Autodesk Fusion 360 part; units mm, degrees
(part 4 of 4)
  line L740 (15.875, 67.5068) -> (19.375, 69.5275)
  line L741 (28.375, 73.569) -> (24.875, 75.5897)
  line L742 (12.375, 69.5275) -> (15.875, 67.5068)
  line L743 (20.375, 59.7125) -> (23.875, 61.7333)
  line L744 (29.375, 67.7955) -> (25.875, 65.7747)
  line L745 (21.375, 73.569) -> (21.375, 69.5275)
  line L746 (16.875, 61.7333) -> (20.375, 59.7125)
  line L747 (25.875, 61.7333) -> (29.375, 59.7125)
  line L748 (25.875, 65.7747) -> (25.875, 61.7333)
  line L749 (23.875, 61.7333) -> (23.875, 65.7747)
  line L750 (16.875, 65.7747) -> (16.875, 61.7333)
  line L751 (32.875, 61.7333) -> (32.875, 65.7747)
  line L752 (15.875, 75.5897) -> (12.375, 73.569)
  line L753 (32.875, 65.7747) -> (29.375, 67.7955)
  line L754 (37.375, 73.569) -> (33.875, 75.5897)
  line L755 (46.375, 69.5275) -> (46.375, 73.569)
  line L756 (42.875, 75.5897) -> (39.375, 73.569)
  line L757 (39.375, 69.5275) -> (42.875, 67.5068)
  line L758 (41.875, 65.7747) -> (38.375, 67.7955)
  line L759 (37.375, 69.5275) -> (37.375, 73.569)
  line L760 (47.375, 59.7125) -> (50.875, 61.7333)
  line L761 (30.375, 73.569) -> (30.375, 69.5275)
  line L762 (42.875, 67.5068) -> (46.375, 69.5275)
  line L763 (38.375, 67.7955) -> (34.875, 65.7747)
  line L764 (33.875, 67.5068) -> (37.375, 69.5275)
  line L765 (46.375, 73.569) -> (42.875, 75.5897)
  line L766 (30.375, 69.5275) -> (33.875, 67.5068)
  line L767 (38.375, 59.7125) -> (41.875, 61.7333)
  line L768 (47.375, 67.7955) -> (43.875, 65.7747)
  line L769 (39.375, 73.569) -> (39.375, 69.5275)
  line L770 (34.875, 61.7333) -> (38.375, 59.7125)
  line L771 (43.875, 61.7333) -> (47.375, 59.7125)
  line L772 (43.875, 65.7747) -> (43.875, 61.7333)
  line L773 (41.875, 61.7333) -> (41.875, 65.7747)
  line L774 (34.875, 65.7747) -> (34.875, 61.7333)
  line L775 (50.875, 61.7333) -> (50.875, 65.7747)
  line L776 (33.875, 75.5897) -> (30.375, 73.569)
  line L777 (50.875, 65.7747) -> (47.375, 67.7955)
  line L778 (55.375, 73.569) -> (51.875, 75.5897)
  line L779 (64.375, 69.5275) -> (64.375, 73.569)
  line L780 (60.875, 75.5897) -> (57.375, 73.569)
  line L781 (57.375, 69.5275) -> (60.875, 67.5068)
  line L782 (59.875, 65.7747) -> (56.375, 67.7955)
  line L783 (55.375, 69.5275) -> (55.375, 73.569)
  line L784 (65.375, 59.7125) -> (68.875, 61.7333)
  line L785 (48.375, 73.569) -> (48.375, 69.5275)
  line L786 (60.875, 67.5068) -> (64.375, 69.5275)
  line L787 (56.375, 67.7955) -> (52.875, 65.7747)
  line L788 (51.875, 67.5068) -> (55.375, 69.5275)
  line L789 (64.375, 73.569) -> (60.875, 75.5897)
  line L790 (48.375, 69.5275) -> (51.875, 67.5068)
  line L791 (56.375, 59.7125) -> (59.875, 61.7333)
  line L792 (65.375, 67.7955) -> (61.875, 65.7747)
  line L793 (57.375, 73.569) -> (57.375, 69.5275)
  line L794 (52.875, 61.7333) -> (56.375, 59.7125)
  line L795 (61.875, 61.7333) -> (65.375, 59.7125)
  line L796 (61.875, 65.7747) -> (61.875, 61.7333)
  line L797 (59.875, 61.7333) -> (59.875, 65.7747)
  line L798 (52.875, 65.7747) -> (52.875, 61.7333)
  line L799 (68.875, 61.7333) -> (68.875, 65.7747)
  line L800 (51.875, 75.5897) -> (48.375, 73.569)
  line L801 (68.875, 65.7747) -> (65.375, 67.7955)
  line L802 (73.375, 73.569) -> (69.875, 75.5897)
  line L803 (82.375, 69.5275) -> (82.375, 73.569)
  line L804 (78.875, 75.5897) -> (75.375, 73.569)
  line L805 (75.375, 69.5275) -> (78.875, 67.5068)
  line L806 (77.875, 65.7747) -> (74.375, 67.7955)
  line L807 (73.375, 69.5275) -> (73.375, 73.569)
  line L808 (83.375, 59.7125) -> (86.875, 61.7333)
  line L809 (66.375, 73.569) -> (66.375, 69.5275)
  line L810 (78.875, 67.5068) -> (82.375, 69.5275)
  line L811 (74.375, 67.7955) -> (70.875, 65.7747)
  line L812 (69.875, 67.5068) -> (73.375, 69.5275)
  line L813 (82.375, 73.569) -> (78.875, 75.5897)
  line L814 (66.375, 69.5275) -> (69.875, 67.5068)
  line L815 (74.375, 59.7125) -> (77.875, 61.7333)
  line L816 (83.375, 67.7955) -> (79.875, 65.7747)
  line L817 (75.375, 73.569) -> (75.375, 69.5275)
  line L818 (70.875, 61.7333) -> (74.375, 59.7125)
  line L819 (79.875, 61.7333) -> (83.375, 59.7125)
  line L820 (79.875, 65.7747) -> (79.875, 61.7333)
  line L821 (77.875, 61.7333) -> (77.875, 65.7747)
  line L822 (70.875, 65.7747) -> (70.875, 61.7333)
  line L823 (86.875, 61.7333) -> (86.875, 65.7747)
  line L824 (69.875, 75.5897) -> (66.375, 73.569)
  line L825 (86.875, 65.7747) -> (83.375, 67.7955)
  line L826 (91.375, 73.569) -> (87.875, 75.5897)
  line L827 (100.375, 69.5275) -> (100.375, 73.569)
  line L828 (96.875, 75.5897) -> (93.375, 73.569)
  line L829 (93.375, 69.5275) -> (96.875, 67.5068)
  line L830 (95.875, 65.7747) -> (92.375, 67.7955)
  line L831 (91.375, 69.5275) -> (91.375, 73.569)
  line L832 (101.375, 59.7125) -> (104.875, 61.7333)
  line L833 (84.375, 73.569) -> (84.375, 69.5275)
  line L834 (96.875, 67.5068) -> (100.375, 69.5275)
  line L835 (92.375, 67.7955) -> (88.875, 65.7747)
  line L836 (87.875, 67.5068) -> (91.375, 69.5275)
  line L837 (100.375, 73.569) -> (96.875, 75.5897)
  line L838 (84.375, 69.5275) -> (87.875, 67.5068)
  line L839 (92.375, 59.7125) -> (95.875, 61.7333)
  line L840 (101.375, 67.7955) -> (97.875, 65.7747)
  line L841 (93.375, 73.569) -> (93.375, 69.5275)
  line L842 (88.875, 61.7333) -> (92.375, 59.7125)
  line L843 (97.875, 61.7333) -> (101.375, 59.7125)
  line L844 (97.875, 65.7747) -> (97.875, 61.7333)
  line L845 (95.875, 61.7333) -> (95.875, 65.7747)
  line L846 (88.875, 65.7747) -> (88.875, 61.7333)
  line L847 (104.875, 61.7333) -> (104.875, 65.7747)
  line L848 (87.875, 75.5897) -> (84.375, 73.569)
  line L849 (104.875, 65.7747) -> (101.375, 67.7955)
  line L850 (109.375, 73.569) -> (105.875, 75.5897)
  line L851 (118.375, 69.5275) -> (118.375, 73.569)
  line L852 (114.875, 75.5897) -> (111.375, 73.569)
  line L853 (111.375, 69.5275) -> (114.875, 67.5068)
  line L854 (113.875, 65.7747) -> (110.375, 67.7955)
  line L855 (109.375, 69.5275) -> (109.375, 73.569)
  line L856 (119.375, 59.7125) -> (122.875, 61.7333)
  line L857 (102.375, 73.569) -> (102.375, 69.5275)
  line L858 (114.875, 67.5068) -> (118.375, 69.5275)
  line L859 (110.375, 67.7955) -> (106.875, 65.7747)
  line L860 (105.875, 67.5068) -> (109.375, 69.5275)
  line L861 (118.375, 73.569) -> (114.875, 75.5897)
  line L862 (102.375, 69.5275) -> (105.875, 67.5068)
  line L863 (110.375, 59.7125) -> (113.875, 61.7333)
  line L864 (119.375, 67.7955) -> (115.875, 65.7747)
  line L865 (111.375, 73.569) -> (111.375, 69.5275)
  line L866 (106.875, 61.7333) -> (110.375, 59.7125)
  line L867 (115.875, 61.7333) -> (119.375, 59.7125)
  line L868 (115.875, 65.7747) -> (115.875, 61.7333)
  line L869 (113.875, 61.7333) -> (113.875, 65.7747)
  line L870 (106.875, 65.7747) -> (106.875, 61.7333)
  line L871 (122.875, 61.7333) -> (122.875, 65.7747)
  line L872 (105.875, 75.5897) -> (102.375, 73.569)
  line L873 (122.875, 65.7747) -> (119.375, 67.7955)
  point P0 (56.375, 32)
  point P1 (65.375, 32)
  point P2 (60.875, 39.7942)
  point P3 (51.875, 39.7942)
  point P4 (11.375, 0.246)
  point P5 (-2.125, 8.0402)
  point P6 (6.875, 8.0402)
  point P7 (2.375, 0.246)
  point P8 (29.375, 0.246)
  point P9 (15.875, 8.0402)
  point P10 (24.875, 8.0402)
  point P11 (20.375, 0.246)
  point P12 (47.375, 0.246)
  point P13 (33.875, 8.0402)
  point P14 (42.875, 8.0402)
  point P15 (38.375, 0.246)
  point P16 (65.375, 0.246)
  point P17 (51.875, 8.0402)
  point P18 (60.875, 8.0402)
  point P19 (56.375, 0.246)
  point P20 (83.375, 0.246)
  point P21 (69.875, 8.0402)
  point P22 (78.875, 8.0402)
  point P23 (74.375, 0.246)
  point P24 (101.375, 0.246)
  point P25 (87.875, 8.0402)
  point P26 (96.875, 8.0402)
  point P27 (92.375, 0.246)
  point P28 (119.375, 0.246)
  point P29 (105.875, 8.0402)
  point P30 (114.875, 8.0402)
  point P31 (110.375, 0.246)
  point P32 (11.375, 16.123)
  point P33 (-2.125, 23.9172)
  point P34 (6.875, 23.9172)
  point P35 (2.375, 16.123)
  point P36 (29.375, 16.123)
  point P37 (15.875, 23.9172)
  point P38 (24.875, 23.9172)
  point P39 (20.375, 16.123)
  point P40 (47.375, 16.123)
  point P41 (33.875, 23.9172)
  point P42 (42.875, 23.9172)
  point P43 (38.375, 16.123)
  point P44 (65.375, 16.123)
  point P45 (51.875, 23.9172)
  point P46 (60.875, 23.9172)
  point P47 (56.375, 16.123)
  point P48 (83.375, 16.123)
  point P49 (69.875, 23.9172)
  point P50 (78.875, 23.9172)
  point P51 (74.375, 16.123)
  point P52 (101.375, 16.123)
  point P53 (87.875, 23.9172)
  point P54 (96.875, 23.9172)
  point P55 (92.375, 16.123)
  point P56 (119.375, 16.123)
  point P57 (105.875, 23.9172)
  point P58 (114.875, 23.9172)
  point P59 (110.375, 16.123)
  point P60 (11.375, 32)
  point P61 (-2.125, 39.7942)
  point P62 (6.875, 39.7942)
  point P63 (2.375, 32)
  point P64 (29.375, 32)
  point P65 (15.875, 39.7942)
  point P66 (24.875, 39.7942)
  point P67 (20.375, 32)
  point P68 (47.375, 32)
  point P69 (33.875, 39.7942)
  point P70 (42.875, 39.7942)
  point P71 (38.375, 32)
  point P72 (83.375, 32)
  point P73 (69.875, 39.7942)
  point P74 (78.875, 39.7942)
  point P75 (74.375, 32)
  point P76 (101.375, 32)
  point P77 (87.875, 39.7942)
  point P78 (96.875, 39.7942)
  point P79 (92.375, 32)
  point P80 (119.375, 32)
  point P81 (105.875, 39.7942)
  point P82 (114.875, 39.7942)
  point P83 (110.375, 32)
  point P84 (11.375, 47.877)
  point P85 (-2.125, 55.6712)
  point P86 (6.875, 55.6712)
  point P87 (2.375, 47.877)
  point P88 (29.375, 47.877)
  point P89 (15.875, 55.6712)
  point P90 (24.875, 55.6712)
  point P91 (20.375, 47.877)
  point P92 (47.375, 47.877)
  point P93 (33.875, 55.6712)
  point P94 (42.875, 55.6712)
  point P95 (38.375, 47.877)
  point P96 (65.375, 47.877)
  point P97 (51.875, 55.6712)
  point P98 (60.875, 55.6712)
  point P99 (56.375, 47.877)
  point P100 (83.375, 47.877)
  point P101 (69.875, 55.6712)
  point P102 (78.875, 55.6712)
  point P103 (74.375, 47.877)
  point P104 (101.375, 47.877)
  point P105 (87.875, 55.6712)
  point P106 (96.875, 55.6712)
  point P107 (92.375, 47.877)
  point P108 (119.375, 47.877)
  point P109 (105.875, 55.6712)
  point P110 (114.875, 55.6712)
  point P111 (110.375, 47.877)
  point P112 (11.375, 63.754)
  point P113 (-2.125, 71.5482)
  point P114 (6.875, 71.5482)
  point P115 (2.375, 63.754)
  point P116 (29.375, 63.754)
  point P117 (15.875, 71.5482)
  point P118 (24.875, 71.5482)
  point P119 (20.375, 63.754)
  point P120 (47.375, 63.754)
  point P121 (33.875, 71.5482)
  point P122 (42.875, 71.5482)
  point P123 (38.375, 63.754)
  point P124 (65.375, 63.754)
  point P125 (51.875, 71.5482)
  point P126 (60.875, 71.5482)
  point P127 (56.375, 63.754)
  point P128 (83.375, 63.754)
  point P129 (69.875, 71.5482)
  point P130 (78.875, 71.5482)
  point P131 (74.375, 63.754)
  point P132 (101.375, 63.754)
  point P133 (87.875, 71.5482)
  point P134 (96.875, 71.5482)
  point P135 (92.375, 63.754)
  point P136 (119.375, 63.754)
  point P137 (105.875, 71.5482)
  point P138 (114.875, 71.5482)
  point P139 (110.375, 63.754)
  dimension "d134" = 6
  dimension "d135" = 2
  dimension "d136" = 54
  dimension "d137" = 2
  dimension "d138" = 2
  dimension "d139" = 3.5
  dimension "d140" = 3.5
  dimension "d141" = 3.5
  dimension "d142" = 3.5
  dimension "d143" = 2
  dimension "d144" = 2
  dimension "d145" = 2
  dimension "d146" = 2
  dimension "d147" = 2
  dimension "d150" = 18
  dimension "d151" = 15.877
  constraint horizontal L16
  constraint vertical L17
  constraint horizontal L18
  constraint vertical L19
  constraint coincident L12.end L13.start
  constraint horizontal L20
  constraint vertical L21
  constraint horizontal L22
  constraint vertical L23
  constraint horizontal L24
  constraint vertical L25
  constraint horizontal L26
  constraint vertical L27
  constraint horizontal L28
  constraint vertical L29
  constraint horizontal L30
  constraint vertical L31
  constraint vertical L32
  constraint horizontal L33
  measures "d134" distance of L12.end L18.end
  measures "d135" distance of L17.end L20.end
  measures "d136" distance of L17.end L22.end
  measures "d137" distance of L22.end L26.end
  measures "d138" distance of L25.end L28.end
  measures "d139" distance of P0 L39
  measures "d140" distance of P1 L45
  measures "d141" distance of P2 L51
  measures "d142" distance of P3 L57
  measures "d143" distance of L39 L42
  measures "d144" distance of L34 L49
  measures "d145" distance of L41 L50
  measures "d146" distance of L48 L57
  measures "d147" distance of L35 L56
extrude "Extrude19" cut sketch "Sketch15" against normal blind 2 contours L18 L33 L178 L183 L185 L188 L190 L200 | L18 L33 L155 L156 L157 L162 L165 L169 | L18 L33 L179 L180 L181 L186 L189 L193 | L18 L33 L154 L159 L161 L164 L166 L176 | L18 L33 L202 L207 L209 L212 L214 L224 | L18 L33 L131 L132 L133 L138 L141 L145 | L18 L29 L32 L33 L204 L205 L217 | L18 L130 L135 L137 L140 L142 L152 | L29 L32 L374 L379 L383 L386 L390 | L18 L107 L108 L109 L114 L117 L121 | L29 L32 L372 L373 L385 | L18 L106 L111 L113 L116 L118 L128 | L29 L516 L517 L529 | L29 L32 L518 L523 L527 L530 L534 | L18 L83 L84 L85 L90 L93 L97 | L26 L29 L684 L685 L697 | L29 L686 L691 L695 L698 L702 | L18 L82 L87 L89 L92 L94 L104 | L26 L682 L687 L689 L692 L694 L704 | L18 L59 L60 L61 L66 L69 L73 | L26 L659 L660 L661 L666 L669 L673 | L18 L21 L58 L63 L68 | L26 L658 L663 L665 L668 L670 L680 | L21 L235 L242 L246 | L21 L230 L235 L239 L242 L245 | L21 L226 L231 L236 | L26 L635 L636 L637 L642 L645 L649 | L21 L394 L399 L404 | L21 L403 L410 L414 | L21 L398 L403 L407 L410 L413 | L26 L634 L639 L641 L644 L646 L656 | L21 L26 L538 L543 L548 | L21 L547 L554 L558 | L21 L542 L547 L551 L554 L557 | L26 L611 L612 L613 L618 L621 L625 | L21 L26 L538 | L26 L610 L615 L617 L620 L622 L632 | L26 L539 L540 L541 L546 L549 L553 | L26 L587 L588 L589 L594 L597 L601 | L26 L562 L567 L569 L572 L574 L584 | L26 L586 L591 L593 L596 L598 L608 | L26 L563 L564 L565 L570 L573 L577 | L34 L35 L36 L37 L38 L39 | L40 L41 L42 L43 L44 L45 | L46 L47 L48 L49 L50 L51 | L52 L53 L54 L55 L56 L57 | L227 L228 L229 L234 L237 L241 | L232 L240 L243 L244 L247 L249 | L250 L255 L257 L260 L262 L272 | L251 L252 L253 L258 L261 L265 | L254 L259 L263 L266 L269 L270 | L256 L264 L267 L268 L271 L273 | L274 L279 L281 L284 L286 L296 | L275 L276 L277 L282 L285 L289 | L278 L283 L287 L290 L293 L294 | L280 L288 L291 L292 L295 L297 | L298 L303 L305 L308 L310 L320 | L299 L300 L301 L306 L309 L313 | L302 L307 L311 L314 L317 L318 | L304 L312 L315 L316 L319 L321 | L322 L327 L329 L332 L334 L344 | L323 L324 L325 L330 L333 L337 | L326 L331 L335 L338 L341 L342 | L328 L336 L339 L340 L343 L345 | L346 L351 L353 L356 L358 L368 | L347 L348 L349 L354 L357 L361 | L350 L355 L359 L362 L365 L366 | L352 L360 L363 L364 L367 L369 | L370 L375 L377 L380 L382 L392 | L395 L396 L397 L402 L405 L409 | L400 L408 L411 L412 L415 L417 | L418 L423 L425 L428 L430 L440 | L419 L420 L421 L426 L429 L433 | L422 L427 L431 L434 L437 L438 | L424 L432 L435 L436 L439 L441 | L442 L447 L449 L452 L454 L464 | L443 L444 L445 L450 L453 L457 | L446 L451 L455 L458 L461 L462 | L448 L456 L459 L460 L463 L465 | L466 L471 L473 L476 L478 L488 | L467 L468 L469 L474 L477 L481 | L470 L475 L479 L482 L485 L486 | L472 L480 L483 L484 L487 L489 | L490 L495 L497 L500 L502 L512 | L491 L492 L493 L498 L501 L505 | L494 L499 L503 L506 L509 L510 | L496 L504 L507 L508 L511 L513 | L514 L519 L521 L524 L526 L536 | L544 L552 L555 L556 L559 L561 | L566 L571 L575 L578 L581 L582 | L568 L576 L579 L580 L583 L585 | L590 L595 L599 L602 L605 L606 | L592 L600 L603 L604 L607 L609 | L614 L619 L623 L626 L629 L630 | L616 L624 L627 L628 L631 L633 | L638 L643 L647 L650 L653 L654 | L640 L648 L651 L652 L655 L657 | L662 L667 L671 L674 L677 L678 | L664 L672 L675 L676 L679 L681 bodies 3
copy_body "CopyPasteBodies1" bodies 2 makes body 4
move_body "Move7" bodies 4 to x (-1, 0, 0) y (0, 1, 0) z (0, 0, -1) at (151, 0, -115)
copy_body "CopyPasteBodies2" bodies 3 makes body 5
move_body "Move8" bodies 5 to x (-1, 0, 0) y (0, 1, 0) z (0, 0, -1) at (151, 0, -115)
equation "d13 = 40 mm + 10 mm + 15 mm"
equation "d14 = 40 mm + 15 mm + 10 mm"
equation "d57 = 20 mm + 9 mm"
equation "d116 = 4.500 mm + 1.5 mm"
named bodies: "Floor", "Long Wall", "Short Wall", "Long Wall (1)", "Short Wall (1)"
